Autodesk Inventor part; units mm, degrees
note: some values were not read from the file. Chosen so that the rebuilt part matches the saved one: direction of "Hole2".
(part 11 of 20)
  ellipse E432 centre (-86.942707, -24.960854) end of major axis (-87.005567, -25.140154) minor radius 0.159857 (-87.101831, -24.938104) -> (-87.104335, -24.953281) ccw
  ellipse E433 centre (-87.045046, -26.985099) end of major axis (-87.107906, -27.1644) minor radius 0.159857 (-87.203438, -27.050403) -> (-87.173284, -27.116116) ccw
  ellipse E434 centre (-86.968538, -27.011922) end of major axis (-86.905679, -26.832621) minor radius 0.159857 (-87.12926, -27.065414) -> (-87.11527, -27.111844) ccw
  ellipse E435 centre (-85.901164, -27.123317) end of major axis (-85.890259, -27.313004) minor radius 0.096916 (-85.84108, -27.281831) -> (-85.804254, -27.157292) ccw
  line L584 (-87.328557, -28.962799) -> (-86.699455, -28.926635)
  line L585 (-86.801552, -28.901283) -> (-87.00211, -28.912813)
  line L586 (-87.352619, -28.932962) -> (-87.409719, -28.936244)
  ellipse E436 centre (-86.50954, -28.967752) end of major axis (-86.259859, -28.980375) minor radius 0.044682 (-86.294863, -28.955411) -> (-86.426351, -28.929641) ccw
  ellipse E437 centre (-86.211464, -23.071891) end of major axis (-86.610953, -23.051694) minor radius 0.071491 (-85.867981, -23.052146) -> (-86.354802, -22.998063) ccw
  ellipse E438 centre (-86.50954, -28.967752) end of major axis (-86.90903, -28.947555) minor radius 0.071491 (-86.166057, -28.948006) -> (-86.535239, -28.895062) ccw
  ellipse E439 centre (-107.037567, -24.524653) end of major axis (-106.979164, -24.705455) minor radius 0.167961 (-107.207727, -24.512455) -> (-107.03633, -24.712285) ccw
  ellipse E440 centre (-107.104293, -24.546207) end of major axis (-107.045891, -24.727009) minor radius 0.167961 (-107.234111, -24.657111) -> (-107.103057, -24.733839) ccw
  ellipse E441 centre (-107.085943, -27.331063) end of major axis (-107.144345, -27.150262) minor radius 0.167961 (-107.144345, -27.150262) -> (-107.207795, -27.190448) ccw
  ellipse E442 centre (-107.293144, -24.539693) end of major axis (-107.306729, -24.729207) minor radius 0.083645 (-107.291907, -24.727325) -> (-107.208623, -24.512391) ccw
  ellipse E443 centre (-107.427481, -24.530063) end of major axis (-107.441066, -24.719577) minor radius 0.083645 (-107.426245, -24.717695) -> (-107.342961, -24.502761) ccw
  ellipse E444 centre (-107.409131, -27.314919) end of major axis (-107.395546, -27.125406) minor radius 0.083645 (-107.32461, -27.287618) -> (-107.410367, -27.127287) ccw
  ellipse E445 centre (-107.019216, -27.309509) end of major axis (-107.077618, -27.128708) minor radius 0.167961 (-107.020452, -27.121877) -> (-107.189377, -27.297312) ccw
  ellipse E446 centre (-107.274793, -27.324549) end of major axis (-107.261208, -27.135035) minor radius 0.083645 (-107.190272, -27.297247) -> (-107.261208, -27.135035) ccw
  line L587 (-107.077618, -27.128708) -> (-107.144345, -27.150262)
  line L588 (-107.261208, -27.135035) -> (-107.395546, -27.125406)
  line L589 (-106.602426, -24.769726) -> (-107.103057, -24.733839)
  line L590 (-107.03633, -24.712285) -> (-106.535699, -24.748172)
  line L591 (-107.702049, -24.806785) -> (-107.688858, -24.802525)
  line L592 (-107.687519, -24.802092) -> (-107.426245, -24.717695)
  line L593 (-107.291907, -24.727325) -> (-107.462106, -24.782303)
  line L594 (-107.410367, -27.127287) -> (-107.564536, -27.177087)
  line L595 (-107.771928, -27.056047) -> (-107.780287, -25.787494)
  line L596 (-107.783195, -25.346207) -> (-107.785333, -25.021719)
  line L597 (-106.763393, -27.140304) -> (-107.020452, -27.121877)
  line L598 (-107.650996, -25.031349) -> (-107.649306, -25.287727)
  line L599 (-107.639861, -26.72106) -> (-107.637591, -27.065677)
  ellipse E447 centre (-107.113404, -23.163654) end of major axis (-107.171806, -22.982853) minor radius 0.167961 (-107.171806, -22.982853) -> (-107.235256, -23.023039) ccw
  ellipse E448 centre (-107.076833, -28.713616) end of major axis (-107.01843, -28.894418) minor radius 0.167961 (-107.20665, -28.82452) -> (-107.075596, -28.901248) ccw
  ellipse E449 centre (-107.010106, -28.692062) end of major axis (-106.951703, -28.872863) minor radius 0.167961 (-107.180267, -28.679864) -> (-107.008869, -28.879694) ccw
  ellipse E450 centre (-107.046677, -23.1421) end of major axis (-107.105079, -22.961299) minor radius 0.167961 (-107.047913, -22.954468) -> (-107.216838, -23.129903) ccw
  line L600 (-107.171806, -22.982853) -> (-107.105079, -22.961299)
  line L601 (-107.075596, -28.901248) -> (-106.888611, -28.914652)
  line L602 (-106.627806, -28.933347) -> (-106.255134, -28.960062)
  line L603 (-107.180267, -28.679864) -> (-107.189377, -27.297312)
  line L604 (-106.832118, -28.892364) -> (-107.008869, -28.879694)
  line L605 (-107.047913, -22.954468) -> (-106.599994, -22.986577)
  line L606 (-107.207727, -24.512455) -> (-107.216838, -23.129903)
  ellipse E451 centre (-106.601189, -24.957359) end of major axis (-106.659592, -24.776557) minor radius 0.167961 (-106.459764, -24.864335) -> (-106.602426, -24.769726) ccw
  ellipse E452 centre (-107.687407, -27.028745) end of major axis (-107.700993, -27.218259) minor radius 0.083645 (-107.771928, -27.056047) -> (-107.760067, -27.145929) ccw
  ellipse E453 centre (-107.700813, -24.994418) end of major axis (-107.687227, -24.804904) minor radius 0.083645 (-107.702049, -24.806785) -> (-107.716578, -24.814285) ccw
  ellipse E454 centre (-107.700813, -24.994418) end of major axis (-107.714398, -25.183931) minor radius 0.083645 (-107.778831, -24.944723) -> (-107.785333, -25.021719) ccw
  ellipse E455 centre (-106.534462, -24.935804) end of major axis (-106.592865, -24.755003) minor radius 0.167961 (-106.480181, -24.762389) -> (-106.535699, -24.748172) ccw
  ellipse E456 centre (-107.55307, -27.038375) end of major axis (-107.539485, -26.848861) minor radius 0.083645 (-107.637591, -27.065677) -> (-107.631847, -27.12943) ccw
  ellipse E457 centre (-107.566475, -25.004047) end of major axis (-107.55289, -24.814534) minor radius 0.083645 (-107.644475, -24.954249) -> (-107.650996, -25.031349) ccw
  line L607 (-107.342961, -24.502761) -> (-107.352071, -23.120209)
  line L608 (-107.437828, -22.959878) -> (-107.663569, -23.032797)
  line L609 (-107.758266, -29.001224) -> (-107.398784, -28.885104)
  line L610 (-107.3155, -28.67017) -> (-107.32461, -27.287618)
  line L611 (-107.208623, -24.512391) -> (-107.217733, -23.129838)
  line L612 (-107.181162, -28.6798) -> (-107.190272, -27.297247)
  line L613 (-108.234209, -29.207986) -> (-107.264446, -28.894734)
  ellipse E458 centre (-107.436591, -23.14751) end of major axis (-107.423006, -22.957997) minor radius 0.083645 (-107.352071, -23.120209) -> (-107.437828, -22.959878) ccw
  ellipse E459 centre (-107.40002, -28.697472) end of major axis (-107.413605, -28.886986) minor radius 0.083645 (-107.398784, -28.885104) -> (-107.3155, -28.67017) ccw
  ellipse E460 centre (-107.302254, -23.15714) end of major axis (-107.288669, -22.967627) minor radius 0.083645 (-107.217733, -23.129838) -> (-107.288669, -22.967627) ccw
  ellipse E461 centre (-107.265683, -28.707102) end of major axis (-107.279268, -28.896616) minor radius 0.083645 (-107.264446, -28.894734) -> (-107.181162, -28.6798) ccw
  line L614 (-107.423006, -22.957997) -> (-107.288669, -22.967627)
  line L615 (-107.998768, -29.268759) -> (-108.121525, -29.259959)
  line L616 (-108.188251, -29.281514) -> (-107.967117, -29.297365)
  ellipse E462 centre (-108.010313, -29.224036) end of major axis (-108.260308, -29.225683) minor radius 0.039312 (-108.234209, -29.207986) -> (-108.121525, -29.259959) ccw
  ellipse E463 centre (-108.010313, -29.224036) end of major axis (-107.610322, -29.2214) minor radius 0.062899 (-108.365264, -29.255315) -> (-108.188251, -29.281514) ccw
  line L617 (-87.436909, -24.723991) -> (-87.336776, -24.724509)
  line L618 (-87.445108, -24.741537) -> (-87.474456, -24.741386)
  line L619 (-87.311646, -26.959148) -> (-87.511604, -24.912298)
  ellipse E464 centre (-87.287323, -23.145711) end of major axis (-87.311854, -22.957301) minor radius 0.092496 (-87.287526, -22.960534) -> (-87.305766, -22.956924) ccw
  ellipse E465 centre (-86.871735, -28.746754) end of major axis (-86.847204, -28.935164) minor radius 0.092496 (-86.853292, -28.935541) -> (-86.847204, -28.935164) ccw
  line L620 (-86.846716, -28.9351) -> (-86.847204, -28.935164)
  line L621 (-87.305766, -22.956924) -> (-87.359069, -22.956648)
  line L622 (-87.292806, -28.915683) -> (-86.989756, -28.917248)
  line L623 (-87.474711, -28.932331) -> (-87.092017, -28.934308)
  line L624 (-86.854297, -28.935536) -> (-86.853292, -28.935541)
  ellipse E466 centre (-87.218509, -26.959629) end of major axis (-87.193977, -27.148039) minor radius 0.092496 (-87.311646, -26.959148) -> (-87.24949, -27.122476) ccw
  ellipse E467 centre (-87.418467, -24.912779) end of major axis (-87.442998, -24.724369) minor radius 0.092496 (-87.436909, -24.723991) -> (-87.511604, -24.912298) ccw
  line L625 (-106.370657, -22.958745) -> (-106.607635, -22.963657)
  line L626 (-106.940274, -28.920181) -> (-106.69829, -28.915165)
  line L627 (-106.832274, -28.937585) -> (-106.577398, -28.932303)
  line L628 (-106.665345, -24.72991) -> (-106.525846, -24.727018)
  line L629 (-106.499131, -25.305468) -> (-106.660854, -26.960927)
  line L630 (-106.490694, -24.745933) -> (-106.53112, -24.746771)
  ellipse E468 centre (-106.544289, -24.915805) end of major axis (-106.52056, -24.727293) minor radius 0.082693 (-106.459145, -24.859035) -> (-106.525846, -24.727018) ccw
  ellipse E469 centre (-106.744247, -26.962656) end of major axis (-106.720518, -26.774144) minor radius 0.082693 (-106.722759, -27.130018) -> (-106.660854, -26.960927) ccw
  ellipse E470 centre (-106.250326, -23.008633) end of major axis (-106.64843, -22.969742) minor radius 0.022991 (-106.607635, -22.963657) -> (-106.64843, -22.969742) ccw
  line L631 (-106.64843, -22.969742) -> (-106.649727, -22.983012)
  line L632 (-85.820471, -29.234615) -> (-85.983673, -29.248237)
  line L633 (-85.979406, -29.27505) -> (-85.746033, -29.255571)
  ellipse E471 centre (-85.819235, -29.046983) end of major axis (-85.870723, -29.229873) minor radius 0.162803 (-85.820471, -29.234615) -> (-85.732823, -29.198768) ccw
  ellipse E472 centre (-85.744796, -29.067939) end of major axis (-85.796285, -29.25083) minor radius 0.162803 (-85.746033, -29.255571) -> (-85.686207, -29.237846) ccw
  line L634 (-86.598662, -24.732341) -> (-86.419734, -24.782714)
  line L635 (-86.217781, -25.02755) -> (-86.231186, -27.061877)
  ellipse E473 centre (-86.945923, -24.761325) end of major axis (-86.545932, -24.76396) minor radius 0.062899 (-86.598662, -24.732341) -> (-87.144426, -24.70544) ccw
  line L636 (-87.345077, -24.722188) -> (-87.144426, -24.70544)
  line L637 (-87.069987, -24.726397) -> (-87.489055, -24.761374)
  ellipse E474 centre (-86.945923, -24.761325) end of major axis (-87.195917, -24.759677) minor radius 0.039312 (-86.728885, -24.74321) -> (-87.069987, -24.726397) ccw
  line L638 (-86.567282, -24.788705) -> (-86.728885, -24.74321)
  line L639 (-87.160304, -27.115032) -> (-87.275182, -27.124621)
  ellipse E475 centre (-86.961801, -27.170916) end of major axis (-87.361792, -27.168281) minor radius 0.062899 (-86.654947, -27.13254) -> (-87.160304, -27.115032) ccw
  line L640 (-86.361408, -27.072746) -> (-86.358434, -26.62133)
  line L641 (-86.351132, -25.513232) -> (-86.348003, -25.038419)
  ellipse E476 centre (-86.31207, -25.001005) end of major axis (-86.327873, -24.811663) minor radius 0.093287 (-86.217781, -25.02755) -> (-86.225725, -24.947506) ccw
  ellipse E477 centre (-86.325475, -27.035332) end of major axis (-86.341278, -26.845991) minor radius 0.093287 (-86.248123, -27.162591) -> (-86.231186, -27.061877) ccw
  ellipse E478 centre (-86.442292, -25.011874) end of major axis (-86.426489, -25.201215) minor radius 0.093287 (-86.348003, -25.038419) -> (-86.352239, -24.979115) ccw
  ellipse E479 centre (-86.455697, -27.046201) end of major axis (-86.439894, -27.235543) minor radius 0.093287 (-86.361679, -27.084661) -> (-86.361408, -27.072746) ccw
  ellipse E480 centre (-86.455697, -27.046201) end of major axis (-86.439894, -27.235543) minor radius 0.093287 (-86.370904, -27.150091) -> (-86.363204, -27.106416) ccw
  line L642 (-86.626123, -28.89975) -> (-86.472854, -28.942899)
  line L643 (-86.756346, -28.910619) -> (-85.674505, -29.215187)
  line L644 (-87.132843, -22.947623) -> (-87.350196, -22.965765)
  ellipse E481 centre (-86.973384, -28.928733) end of major axis (-86.723389, -28.930381) minor radius 0.039312 (-86.756346, -28.910619) -> (-87.090333, -28.893236) ccw
  ellipse E482 centre (-86.93434, -23.003507) end of major axis (-87.334331, -23.000872) minor radius 0.062899 (-86.607298, -22.969394) -> (-87.132843, -22.947623) ccw
  ellipse E483 centre (-86.973384, -28.928733) end of major axis (-87.373375, -28.926098) minor radius 0.062899 (-86.626123, -28.89975) -> (-87.167772, -28.872511) ccw
  ellipse E484 centre (-85.673268, -29.027555) end of major axis (-85.657465, -29.216896) minor radius 0.093287 (-85.674505, -29.215187) -> (-85.657465, -29.216896) ccw
  line L645 (-85.604398, -29.212467) -> (-85.657465, -29.216896)
  ellipse E485 centre (-107.029961, -29.084954) end of major axis (-107.47232, -29.0961) minor radius 0.074077 (-107.192809, -29.020046) -> (-107.256494, -29.026856) ccw
  ellipse E486 centre (-107.179703, -29.04655) end of major axis (-107.029751, -29.042772) minor radius 0.025111 (-107.256494, -29.026856) -> (-107.317709, -29.040104) ccw
  ellipse E487 centre (-107.564096, -29.207458) end of major axis (-107.714049, -29.211237) minor radius 0.025111 (-107.702102, -29.201013) -> (-107.713966, -29.210285) ccw
  ellipse E488 centre (-107.530504, -29.220582) end of major axis (-107.680457, -29.22436) minor radius 0.025111 (-107.657963, -29.236936) -> (-107.655082, -29.237614) ccw
  line L646 (-107.702102, -29.201013) -> (-107.652162, -29.180108)
  line L647 (-107.548659, -29.136781) -> (-107.515543, -29.122918)
  line L648 (-107.344396, -29.051276) -> (-107.317709, -29.040104)
  line L649 (-106.079775, -29.125525) -> (-106.138968, -29.150304)
  ellipse E489 centre (-106.861279, -29.150853) end of major axis (-106.281463, -29.136244) minor radius 0.097095 (-106.880089, -29.05424) -> (-107.323379, -29.103505) ccw
  ellipse E490 centre (-107.355303, -29.06738) end of major axis (-107.205495, -29.059806) minor radius 0.026809 (-107.373403, -29.04162) -> (-107.384849, -29.04251) ccw
  ellipse E491 centre (-107.355303, -29.06738) end of major axis (-107.205495, -29.059806) minor radius 0.026809 (-107.319516, -29.039563) -> (-107.329454, -29.039675) ccw
  ellipse E492 centre (-107.439478, -29.077049) end of major axis (-107.28967, -29.069475) minor radius 0.026809 (-107.512191, -29.057139) -> (-107.575482, -29.072448) ccw
  ellipse E493 centre (-107.851217, -29.256889) end of major axis (-108.001026, -29.264463) minor radius 0.026809 (-107.987221, -29.252288) -> (-107.99809, -29.26937) ccw
  ellipse E494 centre (-107.820239, -29.270455) end of major axis (-107.970048, -29.278029) minor radius 0.026809 (-107.951225, -29.289893) -> (-107.883068, -29.297897) ccw
  line L650 (-108.001731, -29.250516) -> (-108.001026, -29.264463)
  ellipse E495 centre (-107.29769, -29.115875) end of major axis (-107.739625, -29.138218) minor radius 0.079087 (-107.384849, -29.04251) -> (-107.512191, -29.057139) ccw
  ellipse E496 centre (-107.564816, -29.23255) end of major axis (-108.006751, -29.254893) minor radius 0.079087 (-107.99809, -29.26937) -> (-107.951225, -29.289893) ccw
  line L651 (-107.987221, -29.252288) -> (-107.575482, -29.072448)
  line L652 (-107.651638, -29.305727) -> (-107.883068, -29.297897)
  ellipse E497 centre (-107.142135, -29.183994) end of major axis (-107.721395, -29.21328) minor radius 0.103663 (-107.115956, -29.079029) -> (-107.65407, -29.25762) ccw
  ellipse E498 centre (-86.155815, -29.258975) end of major axis (-86.305624, -29.251402) minor radius 0.026809 (-86.079307, -29.285798) -> (-86.018034, -29.276259) ccw
  ellipse E499 centre (-86.133675, -29.244486) end of major axis (-85.983866, -29.252059) minor radius 0.026809 (-85.98454, -29.254338) -> (-86.004869, -29.237081) ccw
  ellipse E500 centre (-86.635055, -29.06871) end of major axis (-86.485247, -29.076284) minor radius 0.026809 (-86.506249, -29.061305) -> (-86.576227, -29.046903) ccw
  ellipse E501 centre (-86.721974, -29.060489) end of major axis (-86.572166, -29.068063) minor radius 0.026809 (-86.79005, -29.033247) -> (-86.798482, -29.033667) ccw
  line L653 (-85.983866, -29.252059) -> (-85.982977, -29.23447)
  ellipse E502 centre (-86.424488, -29.225273) end of major axis (-85.982553, -29.247616) minor radius 0.079087 (-86.018034, -29.276259) -> (-85.98454, -29.254338) ccw
  ellipse E503 centre (-86.749772, -29.111234) end of major axis (-87.191707, -29.088892) minor radius 0.079087 (-86.576227, -29.046903) -> (-86.62803, -29.041071) ccw
  line L654 (-86.506249, -29.061305) -> (-86.004869, -29.237081)
  line L655 (-87.081317, -29.049926) -> (-87.07824, -29.049749)
  line L656 (-86.862818, -29.037365) -> (-86.798482, -29.033667)
  line L657 (-86.079307, -29.285798) -> (-86.351227, -29.301429)
  ellipse E504 centre (-86.860947, -29.183994) end of major axis (-86.281687, -29.21328) minor radius 0.103663 (-86.349012, -29.25762) -> (-86.887126, -29.079029) ccw
  line L658 (-87.985724, -29.229641) -> (-87.864904, -29.270226)
  ellipse E505 centre (-88.474226, -29.415375) end of major axis (-87.896918, -29.359551) minor radius 0.148512 (-87.89795, -29.372979) -> (-87.979459, -29.293773) ccw
  line L659 (-106.138181, -29.269754) -> (-106.01623, -29.218089)
  ellipse E506 centre (-105.528856, -29.415375) end of major axis (-106.106164, -29.359551) minor radius 0.148512 (-106.023623, -29.293773) -> (-106.105133, -29.372979) ccw
  ellipse E507 centre (-106.847411, -29.017366) end of major axis (-106.697414, -29.016378) minor radius 0.023587 (-106.780684, -28.995812) -> (-106.872826, -28.994283) ccw
  ellipse E508 centre (-106.93253, -29.022415) end of major axis (-106.782534, -29.021426) minor radius 0.023587 (-107.001597, -29.00192) -> (-107.066868, -29.012785) ccw
  ellipse E509 centre (-106.79785, -29.062379) end of major axis (-107.24034, -29.065295) minor radius 0.069582 (-106.872826, -28.994283) -> (-107.001597, -29.00192) ccw
  line L660 (-107.136673, -29.035333) -> (-107.066868, -29.012785)
  line L661 (-106.011563, -29.170321) -> (-106.138566, -29.211346)
  line L662 (-106.780684, -28.995812) -> (-105.999982, -29.051776)
  ellipse E510 centre (-106.654122, -29.12867) end of major axis (-106.074135, -29.124848) minor radius 0.091204 (-106.138857, -29.167227) -> (-107.140599, -29.082136) ccw
  ellipse E511 centre (-87.821962, -29.005927) end of major axis (-87.971252, -29.020511) minor radius 0.008622 (-87.691092, -28.997353) -> (-87.685923, -28.996249) ccw
  ellipse E512 centre (-87.821962, -29.005927) end of major axis (-87.971252, -29.020511) minor radius 0.008622 (-87.748433, -29.006306) -> (-87.74616, -29.006009) ccw
  ellipse E513 centre (-87.798086, -28.998604) end of major axis (-87.648797, -28.98402) minor radius 0.008622 (-87.649803, -28.985172) -> (-87.668158, -28.981687) ccw
  line L663 (-87.648797, -28.98402) -> (-87.651481, -28.956542)
  ellipse E514 centre (-88.087239, -29.024797) end of major axis (-87.646835, -28.981774) minor radius 0.025434 (-87.685923, -28.996249) -> (-87.649803, -28.985172) ccw
  line L664 (-88.060773, -28.979659) -> (-87.668158, -28.981687)
  line L665 (-87.748433, -29.006306) -> (-88.004287, -29.039619)
  ellipse E515 centre (-88.519752, -29.059952) end of major axis (-87.9425, -29.00356) minor radius 0.033337 (-88.005702, -29.025142) -> (-88.063098, -28.995) ccw
  line L666 (-106.32881, -28.985153) -> (-105.94269, -28.97715)
  line L667 (-105.998873, -29.040422) -> (-106.231803, -29.011102)
  ellipse E516 centre (-106.194819, -29.002019) end of major axis (-106.344109, -28.987435) minor radius 0.008622 (-106.32881, -28.985153) -> (-106.341842, -28.989209) ccw
  ellipse E517 centre (-106.165966, -29.009737) end of major axis (-106.315256, -28.995153) minor radius 0.008622 (-106.298192, -29.000885) -> (-106.231803, -29.011102) ccw
  line L668 (-106.342419, -28.970142) -> (-106.344109, -28.987435)
  ellipse E518 centre (-105.908125, -29.026999) end of major axis (-106.348529, -28.983976) minor radius 0.025434 (-106.341842, -28.989209) -> (-106.298192, -29.000885) ccw
  ellipse E519 centre (-105.48333, -29.059952) end of major axis (-106.060582, -29.00356) minor radius 0.033337 (-105.939984, -28.995) -> (-105.99738, -29.025142) ccw
  line L669 (-86.980823, -29.008919) -> (-86.8038, -29.058756)
  line L670 (-86.67628, -29.094656) -> (-86.667752, -29.097057)
  line L671 (-88.002732, -29.05554) -> (-87.272127, -28.994561)
  line L672 (-87.864487, -29.206927) -> (-87.991434, -29.171188)
  ellipse E520 centre (-87.111046, -29.019788) end of major axis (-86.961049, -29.020776) minor radius 0.023587 (-86.980823, -29.008919) -> (-87.049852, -28.998645) ccw
  ellipse E521 centre (-87.197688, -29.015517) end of major axis (-87.047692, -29.016505) minor radius 0.023587 (-87.180927, -28.992185) -> (-87.272127, -28.994561) ccw
  ellipse E522 centre (-87.230374, -29.061015) end of major axis (-87.672864, -29.058099) minor radius 0.069582 (-87.049852, -28.998645) -> (-87.180927, -28.992185) ccw
  ellipse E523 centre (-87.34896, -29.12867) end of major axis (-87.928947, -29.124848) minor radius 0.091204 (-86.862483, -29.082136) -> (-87.864225, -29.167227) ccw
  line L673 (-107.583497, -27.119329) -> (-107.609439, -27.130188)
  line L674 (-107.650918, -25.043065) -> (-107.63597, -25.036808)
  line L675 (-107.537495, -27.121477) -> (-107.562128, -27.131788)
  line L676 (-107.583497, -27.119329) -> (-107.586018, -27.019293)
  ellipse E524 centre (-107.488257, -26.97837) end of major axis (-107.476594, -26.728642) minor radius 0.097367 (-107.494466, -26.731976) -> (-107.586018, -27.019293) ccw
  line L677 (-107.494466, -26.731976) -> (-107.144635, -26.585536)
  line L678 (-107.108014, -26.470609) -> (-107.138062, -25.278063)
  line L679 (-107.17965, -25.195875) -> (-107.401033, -25.288546)
  ellipse E525 centre (-107.535689, -25.095921) end of major axis (-107.524025, -24.846193) minor radius 0.097367 (-107.63345, -25.136844) -> (-107.611983, -25.271425) ccw
  line L680 (-107.63345, -25.136844) -> (-107.63597, -25.036808)
  line L681 (-107.09206, -25.280212) -> (-107.062012, -26.472758)
  line L682 (-107.589969, -25.038957) -> (-107.587448, -25.138993)
  ellipse E526 centre (-107.489687, -25.09807) end of major axis (-107.501351, -25.347797) minor radius 0.097367 (-107.587448, -25.138993) -> (-107.572005, -25.253963) ccw
  line L683 (-107.098633, -26.587684) -> (-107.448464, -26.734125)
  ellipse E527 centre (-107.442255, -26.980518) end of major axis (-107.430592, -26.730791) minor radius 0.097367 (-107.448464, -26.734125) -> (-107.540016, -27.021441) ccw
  line L684 (-107.540016, -27.021441) -> (-107.537495, -27.121477)
  line L685 (-107.63597, -25.036808) -> (-107.589969, -25.038957)
  line L686 (-107.537495, -27.121477) -> (-107.583497, -27.119329)
  ellipse E528 centre (-107.147118, -26.486978) end of major axis (-107.151784, -26.586869) minor radius 0.038947 (-107.144635, -26.585536) -> (-107.108014, -26.470609) ccw
  ellipse E529 centre (-107.177167, -25.294432) end of major axis (-107.172501, -25.194541) minor radius 0.038947 (-107.138062, -25.278063) -> (-107.17965, -25.195875) ccw
  ellipse E530 centre (-107.101116, -26.489127) end of major axis (-107.105782, -26.589018) minor radius 0.038947 (-107.098633, -26.587684) -> (-107.062012, -26.472758) ccw
  ellipse E531 centre (-107.131165, -25.296581) end of major axis (-107.126499, -25.19669) minor radius 0.038947 (-107.09206, -25.280212) -> (-107.126499, -25.19669) ccw
  line L687 (-107.172501, -25.194541) -> (-107.126499, -25.19669)
  line L688 (-87.084425, -27.059661) -> (-87.134312, -27.063849)
  line L689 (-87.031952, -24.97714) -> (-87.058988, -24.97941)
  line L690 (-87.127794, -27.073276) -> (-87.05726, -27.067355)
  ellipse E532 centre (-86.873803, -26.793154) end of major axis (-86.805677, -26.552616) minor radius 0.20633 (-87.076736, -26.75449) -> (-87.079549, -26.86613) ccw
  ellipse E533 centre (-86.833896, -25.209335) end of major axis (-86.765769, -24.968796) minor radius 0.20633 (-87.036828, -25.170671) -> (-87.039641, -25.282311) ccw
  spline S43 degree 3 poles (-86.651414, -26.785984) (-86.65205, -26.780163) (-86.653316, -26.76858) (-86.656546, -26.751484) (-86.660694, -26.734784) (-86.665819, -26.718549) (-86.671857, -26.702835) (-86.678776, -26.687702) (-86.686536, -26.673211) (-86.6951, -26.65942) (-86.70443, -26.646389) (-86.714487, -26.634179) (-86.725235, -26.622847) (-86.736637, -26.612458) (-86.748651, -26.603061) (-86.761253, -26.59475) (-86.774361, -26.58747) (-86.783535, -26.583622) (-86.78811, -26.581703) knots 0 0 0 0 0.0680148 0.13532856 0.20193874 0.26783312 0.33299287 0.39739576 0.46101961 0.52384586 0.58586341 0.64707277 0.70749045 0.76715357 0.82612483 0.88449738 0.9423997 1 1 1 1
  spline S44 degree 3 poles (-86.921877, -26.588608) (-86.925867, -26.590633) (-86.933859, -26.59469) (-86.945311, -26.601806) (-86.956355, -26.609628) (-86.966932, -26.618191) (-86.977027, -26.627433) (-86.986618, -26.637317) (-86.99568, -26.647799) (-87.004191, -26.658838) (-87.012129, -26.670392) (-87.01947, -26.682419) (-87.026191, -26.694876) (-87.032269, -26.707723) (-87.037686, -26.720917) (-87.042399, -26.734418) (-87.046455, -26.748173) (-87.048532, -26.757511) (-87.049571, -26.762184) knots 0 0 0 0 0.06018783 0.12057167 0.18123059 0.24222053 0.30357693 0.36531731 0.42744398 0.48994661 0.55280476 0.61599027 0.67946962 0.74320611 0.8071621 0.87130105 0.93558968 1 1 1 1
  spline S45 degree 3 poles (-87.076736, -26.75449) (-87.075541, -26.749883) (-87.07315, -26.740662) (-87.068322, -26.727184) (-87.062644, -26.714007) (-87.056071, -26.701185) (-87.048672, -26.688739) (-87.040487, -26.676701) (-87.031562, -26.665099) (-87.021944, -26.653964) (-87.011678, -26.643325) (-87.000808, -26.633211) (-86.989381, -26.623651) (-86.977441, -26.614677) (-86.965035, -26.606312) (-86.9522, -26.598606) (-86.939011, -26.59152) (-86.929933, -26.587391) (-86.925397, -26.585327) knots 0 0 0 0 0.06075211 0.12157744 0.18258462 0.24385247 0.30543277 0.36735321 0.42962038 0.49222284 0.55513405 0.61831518 0.68171776 0.7452863 0.80896074 0.87267882 0.93637843 1 1 1 1
  spline S46 degree 3 poles (-86.820095, -26.563197) (-86.812871, -26.563511) (-86.798422, -26.564139) (-86.776998, -26.567872) (-86.756238, -26.573705) (-86.736537, -26.581677) (-86.718208, -26.591533) (-86.701304, -26.603118) (-86.685822, -26.616283) (-86.671753, -26.630883) (-86.659092, -26.646776) (-86.647829, -26.66382) (-86.637958, -26.681874) (-86.629471, -26.7008) (-86.622355, -26.720458) (-86.616635, -26.740712) (-86.612183, -26.761413) (-86.610365, -26.775436) (-86.609455, -26.782461) knots 0 0 0 0 0.06486953 0.12974803 0.19473343 0.25817972 0.32016794 0.38123591 0.44183715 0.50233531 0.56300447 0.62403408 0.68553703 0.7475595 0.8100912 0.87307551 0.93641898 1 1 1 1
  spline S47 degree 3 poles (-86.612279, -26.894551) (-86.613529, -26.900817) (-86.615993, -26.913175) (-86.621799, -26.930949) (-86.62901, -26.947718) (-86.637706, -26.963417) (-86.647776, -26.978014) (-86.659162, -26.991467) (-86.671788, -27.003739) (-86.685586, -27.014792) (-86.700483, -27.024589) (-86.716411, -27.033092) (-86.733298, -27.040265) (-86.751076, -27.04607) (-86.769675, -27.050478) (-86.789025, -27.053418) (-86.809062, -27.054983) (-86.822622, -27.054755) (-86.829496, -27.05464) knots 0 0 0 0 0.06465055 0.1274876 0.18889307 0.24923877 0.30888211 0.36816237 0.42739777 0.48688361 0.54689159 0.60767024 0.6694463 0.73242683 0.79680187 0.8627473 0.93042784 1 1 1 1
  spline S48 degree 3 poles (-86.933939, -27.032033) (-86.938624, -27.030022) (-86.947939, -27.026023) (-86.961402, -27.019123) (-86.974345, -27.011633) (-86.986713, -27.003509) (-86.998481, -26.994793) (-87.009619, -26.985502) (-87.020096, -26.975662) (-87.029884, -26.965293) (-87.038951, -26.95442) (-87.047268, -26.943066) (-87.054804, -26.931253) (-87.061529, -26.919005) (-87.067418, -26.906345) (-87.072417, -26.893292) (-87.076584, -26.879887) (-87.078558, -26.870725) (-87.079549, -26.86613) knots 0 0 0 0 0.06647427 0.13218355 0.19716033 0.2614393 0.32505872 0.38806176 0.45049795 0.51242459 0.57390817 0.63502578 0.69586647 0.75653236 0.81713976 0.87781985 0.93871923 1 1 1 1
  spline S49 degree 3 poles (-87.052384, -26.873824) (-87.051772, -26.87728) (-87.050554, -26.884162) (-87.04805, -26.894303) (-87.045084, -26.904234) (-87.041624, -26.913937) (-87.037702, -26.923409) (-87.031886, -26.935698) (-87.023538, -26.950462) (-87.011952, -26.967141) (-86.998933, -26.982675) (-86.984721, -26.997119) (-86.974312, -27.0057) (-86.969111, -27.009988) knots 0 0 0 0 0.0644506 0.12832403 0.1917227 0.2547379 0.31744987 0.37992792 0.50437187 0.62845768 0.75238919 0.87624484 1 1 1 1
  spline S50 degree 3 poles (-86.754789, -27.050292) (-86.751308, -27.048725) (-86.744394, -27.045614) (-86.734582, -27.039952) (-86.7253, -27.033639) (-86.716577, -27.026627) (-86.708403, -27.018959) (-86.700778, -27.010656) (-86.693698, -27.001742) (-86.687163, -26.992241) (-86.681168, -26.982179) (-86.675712, -26.971578) (-86.670791, -26.960463) (-86.666403, -26.948856) (-86.662543, -26.936783) (-86.659221, -26.924264) (-86.656387, -26.91133) (-86.654959, -26.902524) (-86.654238, -26.898073) knots 0 0 0 0 0.05994656 0.11908522 0.17773662 0.23620436 0.29477068 0.35369309 0.41320222 0.47350071 0.53476324 0.59713734 0.66074485 0.72568383 0.79203056 0.85984183 0.92915698 1 1 1 1
  spline S51 degree 3 poles (-86.611506, -25.202165) (-86.612218, -25.195759) (-86.613633, -25.183019) (-86.617365, -25.164255) (-86.622202, -25.145987) (-86.628209, -25.128303) (-86.635303, -25.111281) (-86.643443, -25.095) (-86.652574, -25.07954) (-86.662648, -25.06498) (-86.673614, -25.051401) (-86.685421, -25.038881) (-86.698021, -25.0275) (-86.711363, -25.017343) (-86.725396, -25.008478) (-86.74008, -25.001028) (-86.75533, -24.994927) (-86.7659, -24.992192) (-86.771187, -24.990825) knots 0 0 0 0 0.06847843 0.13617931 0.20309758 0.26921597 0.33450964 0.39895103 0.46251501 0.52518448 0.58695626 0.64784755 0.70790276 0.76720073 0.82586204 0.88405611 0.94200741 1 1 1 1
  spline S52 degree 3 poles (-86.898059, -25.013504) (-86.901542, -25.015689) (-86.908523, -25.020068) (-86.918501, -25.02743) (-86.928118, -25.035346) (-86.937322, -25.043842) (-86.946104, -25.05287) (-86.954446, -25.062403) (-86.96233, -25.072406) (-86.969738, -25.082849) (-86.976653, -25.093699) (-86.983058, -25.104923) (-86.988934, -25.116491) (-86.994263, -25.128369) (-86.999032, -25.140525) (-87.003208, -25.152931) (-87.00683, -25.165542) (-87.008718, -25.174088) (-87.009663, -25.178365) knots 0 0 0 0 0.06025982 0.1207868 0.18162334 0.24279657 0.30432017 0.36619627 0.42841724 0.49096745 0.55382495 0.61696316 0.68035239 0.74396143 0.807759 0.87171523 0.93580312 1 1 1 1
  spline S53 degree 3 poles (-87.036828, -25.170671) (-87.035726, -25.166394) (-87.033521, -25.157836) (-87.029141, -25.1453) (-87.024025, -25.13302) (-87.018128, -25.121038) (-87.011509, -25.109373) (-87.004198, -25.09805) (-86.996234, -25.087092) (-86.987653, -25.076523) (-86.978491, -25.066365) (-86.968784, -25.056643) (-86.958569, -25.04738) (-86.94788, -25.038601) (-86.936758, -25.030325) (-86.925229, -25.022591) (-86.913358, -25.015369) (-86.905168, -25.011043) (-86.901074, -25.008881) knots 0 0 0 0 0.06083705 0.12173396 0.18278727 0.24406937 0.30563053 0.36750102 0.4296934 0.49220474 0.55501884 0.61810841 0.68143706 0.74496132 0.80863248 0.87239845 0.9362055 1 1 1 1
  spline S54 degree 3 poles (-86.801189, -24.980032) (-86.793508, -24.97966) (-86.778169, -24.978918) (-86.755174, -24.980805) (-86.732556, -24.985043) (-86.71079, -24.991831) (-86.690312, -25.000912) (-86.671419, -25.012061) (-86.654129, -25.025085) (-86.638437, -25.039812) (-86.624333, -25.056069) (-86.611808, -25.073686) (-86.600851, -25.092495) (-86.591455, -25.11233) (-86.583602, -25.133025) (-86.57732, -25.154418) (-86.572465, -25.17633) (-86.570521, -25.191194) (-86.569548, -25.198642) knots 0 0 0 0 0.06491361 0.12961858 0.19438015 0.25897481 0.32176837 0.38321901 0.44389655 0.50426715 0.56468953 0.62541836 0.68661292 0.74834873 0.81063045 0.87340478 0.93657257 1 1 1 1
  spline S55 degree 3 poles (-86.572372, -25.310731) (-86.573701, -25.317345) (-86.57632, -25.330379) (-86.582598, -25.349075) (-86.59044, -25.366644) (-86.599926, -25.38301) (-86.61093, -25.398134) (-86.62338, -25.41197) (-86.637189, -25.424471) (-86.652274, -25.435593) (-86.668552, -25.445294) (-86.68594, -25.453528) (-86.704355, -25.460255) (-86.723715, -25.465427) (-86.74394, -25.469011) (-86.764944, -25.470926) (-86.786661, -25.471271) (-86.801289, -25.470077) (-86.808713, -25.469471) knots 0 0 0 0 0.06410082 0.12632292 0.18708858 0.24680768 0.30587245 0.36465307 0.42349429 0.48271369 0.54260125 0.60342049 0.66541057 0.72878933 0.79375677 0.86049868 0.92919035 1 1 1 1
  spline S56 degree 3 poles (-86.912759, -25.43971) (-86.916845, -25.437599) (-86.924975, -25.433399) (-86.936692, -25.426368) (-86.947948, -25.418865) (-86.958691, -25.410851) (-86.968908, -25.402361) (-86.978572, -25.393407) (-86.987662, -25.384007) (-86.996153, -25.374181) (-87.004024, -25.363944) (-87.01125, -25.353315) (-87.01781, -25.342312) (-87.023678, -25.330952) (-87.028837, -25.319254) (-87.033243, -25.307232) (-87.036947, -25.294918) (-87.038741, -25.286522) (-87.039641, -25.282311) knots 0 0 0 0 0.0658533 0.13104018 0.19559045 0.25953687 0.32291608 0.38576964 0.44814503 0.51009667 0.5716869 0.63298697 0.69407787 0.75505117 0.81600962 0.87706766 0.93835167 1 1 1 1
  spline S57 degree 3 poles (-87.012476, -25.290005) (-87.011865, -25.293461) (-87.010647, -25.300342) (-87.008143, -25.310484) (-87.005177, -25.320414) (-87.001717, -25.330118) (-86.997795, -25.339589) (-86.991979, -25.351879) (-86.983631, -25.366643) (-86.972045, -25.383322) (-86.959026, -25.398855) (-86.944813, -25.4133) (-86.934405, -25.42188) (-86.929203, -25.426169) knots 0 0 0 0 0.0644506 0.12832403 0.1917227 0.2547379 0.31744987 0.37992792 0.50437187 0.62845768 0.75238919 0.87624484 1 1 1 1
  spline S58 degree 3 poles (-86.714882, -25.466473) (-86.711401, -25.464906) (-86.704487, -25.461794) (-86.694675, -25.456132) (-86.685393, -25.44982) (-86.67667, -25.442807) (-86.668495, -25.43514) (-86.66087, -25.426836) (-86.653791, -25.417922) (-86.647255, -25.408422) (-86.641261, -25.39836) (-86.635804, -25.387759) (-86.630883, -25.376643) (-86.626496, -25.365037) (-86.622636, -25.352963) (-86.619314, -25.340444) (-86.616479, -25.32751) (-86.615052, -25.318705) (-86.614331, -25.314254) knots 0 0 0 0 0.05994656 0.11908522 0.17773662 0.23620436 0.29477068 0.35369309 0.41320222 0.47350071 0.53476324 0.59713734 0.66074485 0.72568383 0.79203056 0.85984183 0.92915698 1 1 1 1
  ellipse E534 centre (-86.743131, -26.801046) end of major axis (-86.722215, -27.050169) minor radius 0.13482 (-86.612279, -26.894551) -> (-86.609455, -26.782461) ccw
  ellipse E535 centre (-86.78509, -26.804568) end of major axis (-86.806006, -26.555445) minor radius 0.13482 (-86.654238, -26.898073) -> (-86.651414, -26.785984) ccw
  ellipse E536 centre (-86.703224, -25.217226) end of major axis (-86.682308, -25.46635) minor radius 0.13482 (-86.572372, -25.310731) -> (-86.569548, -25.198642) ccw
  ellipse E537 centre (-86.745182, -25.220749) end of major axis (-86.766098, -24.971626) minor radius 0.13482 (-86.614331, -25.314254) -> (-86.611506, -25.202165) ccw
  ellipse E538 centre (-86.846638, -26.800848) end of major axis (-86.914765, -27.041387) minor radius 0.20633 (-87.049571, -26.762184) -> (-87.052384, -26.873824) ccw
  ellipse E539 centre (-86.806731, -25.217029) end of major axis (-86.874858, -25.457567) minor radius 0.20633 (-87.009663, -25.178365) -> (-87.012476, -25.290005) ccw
  ellipse E540 centre (-86.900791, -27.111671) end of major axis (-86.612882, -27.118925) minor radius 0.048213 (-86.883674, -27.063947) -> (-87.05726, -27.067355) ccw
  ellipse E541 centre (-86.900791, -27.111671) end of major axis (-86.612882, -27.118925) minor radius 0.048213 (-86.659109, -27.091379) -> (-86.786758, -27.070179) ccw
  ellipse E542 centre (-86.900791, -27.111671) end of major axis (-87.238683, -27.103157) minor radius 0.056583 (-86.61715, -27.087857) -> (-86.827635, -27.058204) ccw
  ellipse E543 centre (-86.900791, -27.111671) end of major axis (-87.238683, -27.103157) minor radius 0.056583 (-86.956001, -27.054478) -> (-87.084425, -27.059661) ccw
  ellipse E544 centre (-86.848318, -25.02915) end of major axis (-87.18621, -25.020636) minor radius 0.056583 (-86.564677, -25.005336) -> (-86.82786, -24.973154) ccw
  ellipse E545 centre (-86.848318, -25.02915) end of major axis (-87.18621, -25.020636) minor radius 0.056583 (-86.965683, -24.973199) -> (-87.031952, -24.97714) ccw
  line L691 (-86.40513, -27.147906) -> (-86.61715, -27.087857)
  line L692 (-86.564677, -25.005336) -> (-86.533931, -25.014044)
  line L693 (-86.445889, -25.03898) -> (-86.348189, -25.066651)
  line L694 (-86.468936, -27.145241) -> (-86.659109, -27.091379)
  line L695 (-107.747941, -26.746932) -> (-107.422229, -26.604667)
  line L696 (-107.38531, -26.488107) -> (-107.445422, -25.299109)
  line L697 (-107.492276, -25.219139) -> (-107.866994, -25.382809)
  ellipse E546 centre (-107.879414, -25.137148) end of major axis (-107.887867, -25.387005) minor radius 0.10517 (-107.977745, -25.242578) -> (-107.866994, -25.382809) ccw
  line L698 (-107.400088, -25.300643) -> (-107.339976, -26.489641)
  line L699 (-107.376894, -26.6062) -> (-107.703174, -26.748713)
  line L700 (-107.981756, -25.083399) -> (-107.978752, -25.0835)
  ellipse E547 centre (-107.427197, -26.506402) end of major axis (-107.430578, -26.606345) minor radius 0.042068 (-107.422229, -26.604667) -> (-107.38531, -26.488107) ccw
  ellipse E548 centre (-107.487309, -25.317404) end of major axis (-107.483927, -25.217461) minor radius 0.042068 (-107.445422, -25.299109) -> (-107.492276, -25.219139) ccw
  ellipse E549 centre (-107.381862, -26.507936) end of major axis (-107.385243, -26.607879) minor radius 0.042068 (-107.376894, -26.6062) -> (-107.339976, -26.489641) ccw
  ellipse E550 centre (-107.441974, -25.318938) end of major axis (-107.438593, -25.218995) minor radius 0.042068 (-107.400088, -25.300643) -> (-107.438593, -25.218995) ccw
  line L701 (-107.483927, -25.217461) -> (-107.438593, -25.218995)
  ellipse E551 centre (-87.412885, -25.326524) end of major axis (-87.425329, -25.227302) minor radius 0.05049 (-87.399129, -25.237) -> (-87.424089, -25.227177) ccw
  line L702 (-87.424089, -25.227177) -> (-87.480425, -25.231462)
  line L703 (-86.777143, -27.091718) -> (-86.932979, -27.100677)
  line L704 (-86.808226, -27.103912) -> (-86.746446, -27.100361)
  ellipse E552 centre (-86.490128, -26.827333) end of major axis (-86.407418, -26.591411) minor radius 0.210338 (-86.703918, -26.879971) -> (-86.702037, -26.895007) ccw
  ellipse E553 centre (-86.490128, -26.827333) end of major axis (-86.407418, -26.591411) minor radius 0.210338 (-86.69641, -26.783699) -> (-86.702061, -26.812065) ccw
  ellipse E554 centre (-86.410294, -25.248225) end of major axis (-86.327584, -25.012303) minor radius 0.210338 (-86.616575, -25.204591) -> (-86.622203, -25.315899) ccw
  spline S59 degree 3 poles (-86.366638, -26.643184) (-86.369976, -26.640669) (-86.376627, -26.635658) (-86.387197, -26.629057) (-86.398123, -26.623218) (-86.409432, -26.618238) (-86.421092, -26.614139) (-86.433086, -26.610962) (-86.445393, -26.608743) (-86.457993, -26.607521) (-86.470866, -26.607333) (-86.48399, -26.608215) (-86.497313, -26.610199) (-86.510655, -26.613274) (-86.523828, -26.617388) (-86.536658, -26.622489) (-86.54915, -26.628455) (-86.557105, -26.633146) (-86.56109, -26.635496) knots 0 0 0 0 0.06027236 0.12008459 0.17956335 0.23886314 0.2981675 0.35768957 0.41767151 0.47838294 0.54011829 0.60319317 0.66794006 0.7342313 0.80052522 0.86682566 0.93327954 1 1 1 1
  spline S60 degree 3 poles (-86.65611, -26.748206) (-86.657618, -26.751803) (-86.660636, -26.759001) (-86.664553, -26.770047) (-86.668054, -26.781249) (-86.669956, -26.788841) (-86.670907, -26.79264) knots 0 0 0 0 0.24945299 0.49932153 0.74952532 1 1 1 1
  spline S61 degree 3 poles (-86.69641, -26.783699) (-86.695523, -26.780581) (-86.693748, -26.774342) (-86.6905, -26.765159) (-86.686844, -26.756118) (-86.68275, -26.747239) (-86.678247, -26.738528) (-86.67334, -26.73) (-86.668075, -26.721641) (-86.664269, -26.716253) (-86.662362, -26.713553) knots 0 0 0 0 0.12403661 0.24815991 0.37248981 0.49712476 0.62214288 0.74760322 0.87354721 1 1 1 1
  spline S62 degree 3 poles (-86.585113, -26.642376) (-86.580618, -26.639671) (-86.571628, -26.634263) (-86.557623, -26.627087) (-86.543301, -26.620636) (-86.528675, -26.615007) (-86.513812, -26.610217) (-86.498763, -26.606304) (-86.483583, -26.603299) (-86.468327, -26.601237) (-86.453049, -26.600151) (-86.437804, -26.600076) (-86.422646, -26.601045) (-86.407631, -26.603094) (-86.392811, -26.60625) (-86.378334, -26.610554) (-86.364334, -26.615851) (-86.35547, -26.620255) (-86.351084, -26.622434) knots 0 0 0 0 0.06405989 0.1281006 0.19204727 0.25582983 0.3193861 0.38266496 0.44562961 0.50826114 0.57056212 0.63256041 0.69431295 0.75590946 0.81747579 0.87917562 0.94021367 1 1 1 1
  spline S63 degree 3 poles (-86.363417, -27.080287) (-86.367834, -27.081626) (-86.37675, -27.084329) (-86.390556, -27.0873) (-86.40478, -27.089509) (-86.419421, -27.090859) (-86.434446, -27.091358) (-86.449829, -27.090986) (-86.46554, -27.08973) (-86.481555, -27.087575) (-86.497837, -27.084505) (-86.514217, -27.080559) (-86.530435, -27.075731) (-86.546237, -27.070064) (-86.561529, -27.063616) (-86.576256, -27.056394) (-86.590431, -27.048501) (-86.599414, -27.042599) (-86.603881, -27.039665) knots 0 0 0 0 0.0549764 0.11096338 0.16806833 0.22639244 0.28603139 0.34707614 0.40961367 0.47372767 0.53949927 0.6069434 0.67436537 0.7409998 0.80686402 0.87197412 0.93634658 1 1 1 1
  spline S64 degree 3 poles (-86.672638, -26.969926) (-86.674422, -26.96705) (-86.677986, -26.961308) (-86.682804, -26.952397) (-86.687208, -26.943298) (-86.691148, -26.933997) (-86.694626, -26.924509) (-86.697615, -26.91484) (-86.70015, -26.905006) (-86.701407, -26.898345) (-86.702037, -26.895007) knots 0 0 0 0 0.12529925 0.25024005 0.37494166 0.49953681 0.62417216 0.7490086 0.87422136 1 1 1 1
  spline S65 degree 3 poles (-86.676535, -26.903948) (-86.676246, -26.905888) (-86.675671, -26.909759) (-86.674591, -26.915516) (-86.673358, -26.921214) (-86.671961, -26.92685) (-86.670408, -26.932422) (-86.668696, -26.937928) (-86.666844, -26.943372) (-86.665482, -26.946949) (-86.664802, -26.948736) knots 0 0 0 0 0.12682999 0.25300914 0.37860655 0.50368723 0.62831214 0.75253809 0.87641783 1 1 1 1
  spline S66 degree 3 poles (-86.382371, -27.08885) (-86.380628, -27.088131) (-86.377157, -27.086698) (-86.372089, -27.084288) (-86.367144, -27.081718) (-86.363953, -27.079839) (-86.362363, -27.078902) knots 0 0 0 0 0.25282857 0.50351543 0.75244628 1 1 1 1
  spline S67 degree 3 poles (-86.351592, -25.032404) (-86.354714, -25.031732) (-86.360982, -25.030383) (-86.370568, -25.029103) (-86.380312, -25.028378) (-86.390217, -25.028278) (-86.400271, -25.028807) (-86.410466, -25.029985) (-86.420758, -25.031821) (-86.431038, -25.034299) (-86.441198, -25.037391) (-86.451159, -25.041063) (-86.460908, -25.045293) (-86.470431, -25.05006) (-86.479718, -25.055341) (-86.488748, -25.061124) (-86.497537, -25.067353) (-86.50314, -25.071868) (-86.505948, -25.07413) knots 0 0 0 0 0.05778221 0.11602992 0.17490487 0.23457915 0.29523385 0.35705764 0.42024514 0.48436692 0.54838884 0.61238964 0.67645987 0.74067474 0.80509501 0.86976792 0.93472837 1 1 1 1
  spline S68 degree 3 poles (-86.616575, -25.204591) (-86.61627, -25.203478) (-86.61566, -25.201253) (-86.614668, -25.197937) (-86.613626, -25.194636) (-86.612882, -25.192451) (-86.61251, -25.191358) knots 0 0 0 0 0.24996578 0.49993063 0.74993068 1 1 1 1
  spline S69 degree 3 poles (-86.530145, -25.080618) (-86.523495, -25.075702) (-86.510183, -25.065858) (-86.488712, -25.053315) (-86.466361, -25.042517) (-86.443221, -25.03375) (-86.419538, -25.027101) (-86.399472, -25.023441) (-86.383364, -25.021714) (-86.371305, -25.02105) (-86.359268, -25.02097) (-86.351278, -25.021469) (-86.347289, -25.021719) knots 0 0 0 0 0.12626187 0.25278671 0.37919835 0.50514032 0.63031299 0.75451273 0.81623998 0.87771389 0.93895544 1 1 1 1
  spline S70 degree 3 poles (-86.349785, -25.51204) (-86.358213, -25.512006) (-86.370983, -25.511955) (-86.388104, -25.510297) (-86.401275, -25.508494) (-86.414632, -25.506057) (-86.432629, -25.501997) (-86.454778, -25.4955) (-86.480283, -25.485425) (-86.504314, -25.473308) (-86.52303, -25.461524) (-86.537111, -25.451239) (-86.543756, -25.445719) (-86.547064, -25.442971) knots 0 0 0 0 0.11836757 0.17935651 0.24161124 0.30518476 0.370129 0.50087366 0.62916185 0.75504201 0.87860366 0.93956774 1 1 1 1
  spline S71 degree 3 poles (-86.617912, -25.334962) (-86.618336, -25.333394) (-86.619184, -25.330256) (-86.620308, -25.325505) (-86.621331, -25.320721) (-86.621912, -25.317508) (-86.622203, -25.315899) knots 0 0 0 0 0.24922132 0.49890182 0.74913063 1 1 1 1
  ellipse E555 centre (-86.464626, -26.836274) end of major axis (-86.547336, -27.072195) minor radius 0.210338 (-86.670907, -26.79264) -> (-86.677457, -26.827585) ccw
  ellipse E556 centre (-86.464626, -26.836274) end of major axis (-86.547336, -27.072195) minor radius 0.210338 (-86.678958, -26.882459) -> (-86.676535, -26.903948) ccw
  ellipse E557 centre (-86.539394, -27.148401) end of major axis (-86.251762, -27.162943) minor radius 0.051474 (-86.645263, -27.095301) -> (-86.684819, -27.096819) ccw
  ellipse E558 centre (-86.539394, -27.148401) end of major axis (-86.251762, -27.162943) minor radius 0.051474 (-86.364336, -27.116074) -> (-86.577878, -27.095444) ccw
  ellipse E559 centre (-86.539394, -27.148401) end of major axis (-86.876963, -27.131335) minor radius 0.06041 (-86.358617, -27.106167) -> (-86.607387, -27.085829) ccw
  ellipse E560 centre (-86.539394, -27.148401) end of major axis (-86.876963, -27.131335) minor radius 0.06041 (-86.67843, -27.086481) -> (-86.7096, -27.087838) ccw
  ellipse E561 centre (-86.434422, -25.072076) end of major axis (-86.771991, -25.05501) minor radius 0.06041 (-86.348431, -25.017794) -> (-86.549675, -25.009585) ccw
  line L705 (-85.361042, -27.091552) -> (-85.056724, -27.19824)
  line L706 (-85.000751, -27.117858) -> (-84.940639, -25.928859)
  line L707 (-84.986677, -25.812713) -> (-85.290994, -25.706025)
  line L708 (-85.09966, -27.200709) -> (-85.361912, -27.108767)
  ellipse E562 centre (-85.051757, -27.099976) end of major axis (-85.046017, -27.199811) minor radius 0.051008 (-85.056724, -27.19824) -> (-85.000751, -27.117858) ccw
  ellipse E563 centre (-84.991645, -25.910978) end of major axis (-84.997384, -25.811142) minor radius 0.051008 (-84.940639, -25.928859) -> (-84.986677, -25.812713) ccw
  ellipse E564 centre (-85.094692, -27.102444) end of major axis (-85.088953, -27.202279) minor radius 0.051008 (-85.09966, -27.200709) -> (-85.088953, -27.202279) ccw
  line L709 (-85.046017, -27.199811) -> (-85.088953, -27.202279)
  line L710 (-107.288024, -27.083795) -> (-107.334336, -27.098755)
  line L711 (-107.468015, -25.050827) -> (-107.301774, -24.997128)
  line L712 (-107.243245, -27.087005) -> (-107.286532, -27.100988)
  line L713 (-107.288024, -27.083795) -> (-107.288685, -26.98356)
  ellipse E565 centre (-107.177473, -26.947637) end of major axis (-107.159598, -26.698277) minor radius 0.110059 (-107.1791, -26.700752) -> (-107.288685, -26.98356) ccw
  line L714 (-107.1791, -26.700752) -> (-106.781137, -26.572202)
  line L715 (-106.737303, -26.459079) -> (-106.745177, -25.264159)
  line L716 (-106.790312, -25.179774) -> (-107.092152, -25.277274)
  ellipse E566 centre (-107.189902, -25.06144) end of major axis (-107.172027, -24.81208) minor radius 0.110059 (-107.301114, -25.097363) -> (-107.278328, -25.237182) ccw
  line L717 (-107.301114, -25.097363) -> (-107.301774, -24.997128)
  line L718 (-106.700398, -25.267368) -> (-106.692524, -26.462289)
  line L719 (-107.256995, -25.000338) -> (-107.256334, -25.100573)
  ellipse E567 centre (-107.145123, -25.06465) end of major axis (-107.162998, -25.31401) minor radius 0.110059 (-107.256334, -25.100573) -> (-107.240046, -25.221156) ccw
  line L720 (-106.736357, -26.575412) -> (-107.134321, -26.703962)
  ellipse E568 centre (-107.132694, -26.950847) end of major axis (-107.114819, -26.701486) minor radius 0.110059 (-107.134321, -26.703962) -> (-107.243905, -26.98677) ccw
  line L721 (-107.243905, -26.98677) -> (-107.243245, -27.087005)
  line L722 (-107.301774, -24.997128) -> (-107.256995, -25.000338)
  line L723 (-107.243245, -27.087005) -> (-107.288024, -27.083795)
  ellipse E569 centre (-106.781787, -26.473448) end of major axis (-106.788937, -26.573193) minor radius 0.044024 (-106.781137, -26.572202) -> (-106.737303, -26.459079) ccw
  ellipse E570 centre (-106.789661, -25.278528) end of major axis (-106.782511, -25.178784) minor radius 0.044024 (-106.745177, -25.264159) -> (-106.790312, -25.179774) ccw
  ellipse E571 centre (-106.737008, -26.476658) end of major axis (-106.744158, -26.576402) minor radius 0.044024 (-106.736357, -26.575412) -> (-106.692524, -26.462289) ccw
  ellipse E572 centre (-106.744882, -25.281738) end of major axis (-106.737732, -25.181994) minor radius 0.044024 (-106.700398, -25.267368) -> (-106.737732, -25.181994) ccw
  line L724 (-106.782511, -25.178784) -> (-106.737732, -25.181994)